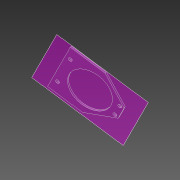
# Autodesk Inventor part: ballcover
Saved by Autodesk Inventor 2018 (Build 220112000, 112)
## iProperties
Created: 2018-07-05
Part Number: ballcover
Material: アルミニウム 6061
Document SubType Name: Modeling
Designer: NaMACHAN
Density: 2.7 g/cm^3
Appearance: アルミニウム - フラット
Mass: 3.92756 g
Surface Area: 24.2056 cm^2
Volume: 1.45465 cm^3
Author: NaMACHAN
Autodesk Inventor part; units mm, degrees
ref_plane "YZ Plane" through (0, 0, 0) normal (1, 0, 0) x (0, 1, 0)
ref_plane "XZ Plane" through (0, 0, 0) normal (0, 1, 0) x (-1, 0, 0)
ref_plane "作業平面2" through (3.9153, -1.6711, -82.7275) normal (-0.2409436, 0.962964, 0.1210227) x (-0.8605128, -0.2696299, 0.4322238)
sketch "スケッチ1" plane through (3.9153, -1.6711, -82.7275) normal (-0.2409436, 0.962964, 0.1210227) x (-0.8605128, -0.2696299, 0.4322238)
  arc A0 (-22.541, -2) -> (2.5598, -16.4919) centre (-4.6524, 0) ccw projected
  line L0 (-7.6524, -23) -> (-29.6524, -6) projected
  line L1 (-29.6524, -6) -> (-29.6524, 6) projected
  line L2 (-29.6524, 6) -> (-7.6524, 23) projected
  line L3 (20.3476, 23) -> (-7.6524, 23) projected
  line L4 (20.3476, 23) -> (20.3476, -23) projected
  line L5 (-7.6524, -23) -> (20.3476, -23) projected
  circle A1 centre (16.3476, 13) radius 1.5 projected
  circle A2 centre (16.3476, -13) radius 1.5 projected
  circle A3 centre (-26.6524, -5) radius 1.5 projected
  circle A4 centre (-26.6524, 5) radius 1.5 projected
  circle A5 centre (-4.6524, 0) radius 16.85
  point P0 (38.6754, 72.1686)
  dimension "d0" = 33.7
  constraints: 1 centre point, 1 coincident
  measures "d0" diameter of A5
extrude "押し出し1" add sketch "スケッチ1" along normal blind 1.5
chamfer "面取り1" distance 1 angle 45 1 edges at (22.4184, 4.1266, -92.0214)
